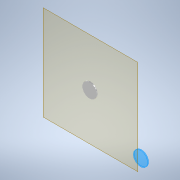
# Autodesk Inventor part: pcb
Saved by Autodesk Inventor 2021 (Build 250183000, 183)
## iProperties
Created: 2023-11-23
Part Number: pcb
Material: Aluminum 6061
Document SubType Name: Modeling
Designer: M
Mass: 34 g
Surface Area: 126.669 cm^2
Volume: 33.2506 cm^3
Density: 1.02254 g/cm^3
Appearance: Aluminum - Flat
Author: M
Autodesk Inventor part; units mm, degrees
ref_plane "YZ Plane" through (0, 0, 0) normal (1, 0, 0) x (0, 1, 0)
ref_plane "XZ Plane" through (0, 0, 0) normal (0, 1, 0) x (-1, 0, 0)
ref_plane "XY Plane" through (0, 0, 0) normal (0, 0, 1) x (1, 0, 0)
ref_plane "Work Plane1" through (0, 0, 0) normal (0, 0, 1) x (1, 0, 0)
sketch "Sketch1" plane through (0, 0, 0) normal (0, 0, 1) x (1, 0, 0)
  circle A0 centre (-243.2728, 252.8536) radius 42
  dimension "d1" = 84
  constraints: 1 centre point, 1 coincident
  measures "d1" diameter of A0
extrude "Extrusion1" add sketch "Sketch1" along normal blind 6
body "Solid1"
